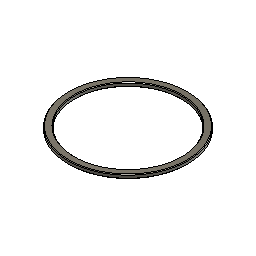
Washer_motor_coupling (Autodesk Fusion 360 design; units mm, degrees)
part number: 2025-04-25-16-45-21-676
Autodesk Fusion 360 part; units mm, degrees
sketch "Sketch1" plane through (0, 0, 0) normal (0, 1, 0) x (1, 0, 0)
  circle A0 centre (0, 0) radius 20
  circle A1 centre (0, 0) radius 22.5
  dimension "d1" = 45
  constraint coincident A0.centre A1.centre
  constraint concentric A0 A1
  measures "d1" diameter of A1
extrude "Extrude1" add sketch "Sketch1" along normal blind 1.5
chamfer "Chamfer1" distance 0.25 angle 45 4 edges at (-18.6465, 1.5, -7.2323) (-18.6465, 0, -7.2323) (-20.9774, 1.5, 8.1363) (-20.9774, 0, 8.1363)
